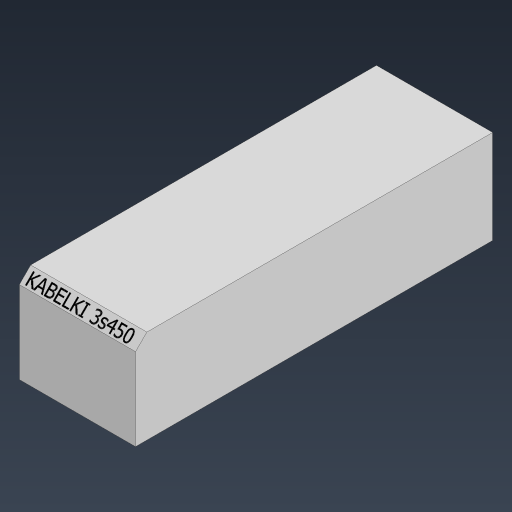
# Autodesk Inventor part: 2s450mah
Saved by Autodesk Inventor 2026.2 (Build 302298010, 298A)
## iProperties
Created: 2026-03-09
Part Number: 2s450mah
Material: Generic
Document SubType Name: Modeling
Designer: szymo
Density: 1 g/cm^3
Appearance: Default
Author: szymo
Autodesk Inventor part; units mm, degrees
ref_plane "YZ Plane" through (0, 0, 0) normal (1, 0, 0) x (0, 1, 0)
ref_plane "XZ Plane" through (0, 0, 0) normal (0, 1, 0) x (-1, 0, 0)
ref_plane "XY Plane" through (0, 0, 0) normal (0, 0, 1) x (1, 0, 0)
sketch "Sketch1" plane through (0, 0, 0) normal (0, 1, 0) x (-1, 0, 0)
  line L0 (0, 0) -> (-20.5, 0)
  line L1 (-20.5, 0) -> (-20.5, -63)
  line L2 (-20.5, -63) -> (0, -63)
  line L3 (0, -63) -> (0, 0)
  dimension "d0" = 20.5
  dimension "d1" = 63
  constraints: 8 end point, 2 parallel, 1 horizontal, 1 perpendicular
  measures "d0" distance of L2.end L1.end
  measures "d1" distance of L0.end L1.end
extrude "Extrusion1" add sketch "Sketch1" along normal blind 16.5
chamfer "Chamfer1" distance 2 angle 45 1 edges at (10.25, 16.5, 0)
sketch "Sketch2" plane through (0, 16.5, -2) normal (0, 0.7071068, 0.7071068) x (1, 0, 0)
  line L0 (0.6017, -0.4664) -> (21.0819, -0.4664) construction
  line L1 (21.0819, -0.4664) -> (21.0819, -2.9145) construction
  line L2 (21.0819, -2.9145) -> (0.6017, -2.9145) construction
  line L3 (0.6017, -2.9145) -> (0.6017, -0.4664) construction
  line L4 (2.263, -2.5085) -> (1.9178, -2.5085)
  line L5 (1.9178, -2.5085) -> (1.1868, -1.5782)
  line L6 (1.1868, -1.5782) -> (1.0701, -1.7095)
  line L7 (1.0701, -1.7095) -> (1.0701, -2.5085)
  line L8 (1.0701, -2.5085) -> (0.8043, -2.5085)
  line L9 (0.8043, -2.5085) -> (0.8043, -0.5085)
  line L10 (0.8043, -0.5085) -> (1.0701, -0.5085)
  line L11 (1.0701, -0.5085) -> (1.0701, -1.4275)
  line L12 (1.0701, -1.4275) -> (1.8902, -0.5085)
  line L13 (1.8902, -0.5085) -> (2.2144, -0.5085)
  line L14 (2.2144, -0.5085) -> (1.3862, -1.4015)
  line L15 (1.3862, -1.4015) -> (2.263, -2.5085)
  line L16 (2.2063, -2.5085) -> (2.8805, -0.5085)
  line L17 (2.8805, -0.5085) -> (3.2079, -0.5085)
  line L18 (3.2079, -0.5085) -> (3.8821, -2.5085)
  line L19 (3.8821, -2.5085) -> (3.6017, -2.5085)
  line L20 (3.6017, -2.5085) -> (3.4202, -1.9493)
  line L21 (3.4202, -1.9493) -> (2.6568, -1.9493)
  line L22 (2.6568, -1.9493) -> (2.4753, -2.5085)
  line L23 (2.4753, -2.5085) -> (2.2063, -2.5085)
  line L24 (3.3473, -1.7224) -> (3.0377, -0.7808)
  line L25 (3.0377, -0.7808) -> (2.7298, -1.7224)
  line L26 (2.7298, -1.7224) -> (3.3473, -1.7224)
  spline S0 degree 2 poles (5.4283, -1.8942) (5.4283, -2.0433) (5.3148, -2.2719) (5.2208, -2.3464) knots 0 0 0 1 2 2 2
  spline S1 degree 2 poles (5.2208, -2.3464) (5.1074, -2.4339) (4.8497, -2.5085) (4.6455, -2.5085) knots 0 0 0 1 2 2 2
  line L27 (4.6455, -2.5085) -> (4.0717, -2.5085)
  line L28 (4.0717, -2.5085) -> (4.0717, -0.5085)
  line L29 (4.0717, -0.5085) -> (4.6017, -0.5085)
  spline S2 degree 2 poles (4.6017, -0.5085) (4.8157, -0.5085) (5.0296, -0.5361) (5.1268, -0.5895) knots 0 0 0 1 2 2 2
  spline S3 degree 2 poles (5.1268, -0.5895) (5.2354, -0.6463) (5.3343, -0.8327) (5.3343, -0.9591) knots 0 0 0 1 2 2 2
  spline S4 degree 2 poles (5.3343, -0.9591) (5.3343, -1.1001) (5.1852, -1.3237) (5.0539, -1.3869) knots 0 0 0 1 2 2 2
  line L30 (5.0539, -1.3869) -> (5.0539, -1.3967)
  spline S5 degree 2 poles (5.0539, -1.3967) (5.2322, -1.4453) (5.4283, -1.703) (5.4283, -1.8942) knots 0 0 0 1 2 2 2
  spline S6 degree 2 poles (5.1512, -1.9056) (5.1512, -1.7921) (5.0863, -1.6463) (4.9891, -1.5944) knots 0 0 0 1 2 2 2
  spline S7 degree 2 poles (4.9891, -1.5944) (4.9259, -1.562) (4.7768, -1.5425) (4.639, -1.5425) knots 0 0 0 1 2 2 2
  line L31 (4.639, -1.5425) -> (4.3375, -1.5425)
  line L32 (4.3375, -1.5425) -> (4.3375, -2.2816)
  line L33 (4.3375, -2.2816) -> (4.5531, -2.2816)
  spline S8 degree 2 poles (4.5531, -2.2816) (4.7281, -2.2816) (4.9291, -2.2492) (5.0069, -2.1973) knots 0 0 0 1 2 2 2
  spline S9 degree 2 poles (5.0069, -2.1973) (5.0815, -2.1438) (5.1512, -2.0109) (5.1512, -1.9056) knots 0 0 0 1 2 2 2
  spline S10 degree 2 poles (5.0571, -0.9963) (5.0571, -0.925) (5.0085, -0.8181) (4.955, -0.7873) knots 0 0 0 1 2 2 2
  spline S11 degree 2 poles (4.955, -0.7873) (4.8902, -0.7516) (4.733, -0.7354) (4.592, -0.7354) knots 0 0 0 1 2 2 2
  line L34 (4.592, -0.7354) -> (4.3375, -0.7354)
  line L35 (4.3375, -0.7354) -> (4.3375, -1.3205)
  line L36 (4.3375, -1.3205) -> (4.639, -1.3205)
  spline S12 degree 2 poles (4.639, -1.3205) (4.7638, -1.3205) (4.8821, -1.2946) (4.9453, -1.254) knots 0 0 0 1 2 2 2
  spline S13 degree 2 poles (4.9453, -1.254) (5.0069, -1.2151) (5.0571, -1.0903) (5.0571, -0.9963) knots 0 0 0 1 2 2 2
  line L37 (5.6925, -2.5085) -> (5.6925, -0.5085)
  line L38 (5.6925, -0.5085) -> (6.9437, -0.5085)
  line L39 (6.9437, -0.5085) -> (6.9437, -0.7451)
  line L40 (6.9437, -0.7451) -> (5.9583, -0.7451)
  line L41 (5.9583, -0.7451) -> (5.9583, -1.2929)
  line L42 (5.9583, -1.2929) -> (6.8772, -1.2929)
  line L43 (6.8772, -1.2929) -> (6.8772, -1.5296)
  line L44 (6.8772, -1.5296) -> (5.9583, -1.5296)
  line L45 (5.9583, -1.5296) -> (5.9583, -2.2719)
  line L46 (5.9583, -2.2719) -> (6.9437, -2.2719)
  line L47 (6.9437, -2.2719) -> (6.9437, -2.5085)
  line L48 (6.9437, -2.5085) -> (5.6925, -2.5085)
  line L49 (8.3943, -2.5085) -> (7.2354, -2.5085)
  line L50 (7.2354, -2.5085) -> (7.2354, -0.5085)
  line L51 (7.2354, -0.5085) -> (7.5012, -0.5085)
  line L52 (7.5012, -0.5085) -> (7.5012, -2.2719)
  line L53 (7.5012, -2.2719) -> (8.3943, -2.2719)
  line L54 (8.3943, -2.2719) -> (8.3943, -2.5085)
  line L55 (10.062, -2.5085) -> (9.7168, -2.5085)
  line L56 (9.7168, -2.5085) -> (8.9858, -1.5782)
  line L57 (8.9858, -1.5782) -> (8.8691, -1.7095)
  line L58 (8.8691, -1.7095) -> (8.8691, -2.5085)
  line L59 (8.8691, -2.5085) -> (8.6033, -2.5085)
  line L60 (8.6033, -2.5085) -> (8.6033, -0.5085)
  line L61 (8.6033, -0.5085) -> (8.8691, -0.5085)
  line L62 (8.8691, -0.5085) -> (8.8691, -1.4275)
  line L63 (8.8691, -1.4275) -> (9.6892, -0.5085)
  line L64 (9.6892, -0.5085) -> (10.0134, -0.5085)
  line L65 (10.0134, -0.5085) -> (9.1852, -1.4015)
  line L66 (9.1852, -1.4015) -> (10.062, -2.5085)
  line L67 (10.9178, -2.5085) -> (10.143, -2.5085)
  line L68 (10.143, -2.5085) -> (10.143, -2.3043)
  line L69 (10.143, -2.3043) -> (10.3975, -2.3043)
  line L70 (10.3975, -2.3043) -> (10.3975, -0.7127)
  line L71 (10.3975, -0.7127) -> (10.143, -0.7127)
  line L72 (10.143, -0.7127) -> (10.143, -0.5085)
  line L73 (10.143, -0.5085) -> (10.9178, -0.5085)
  line L74 (10.9178, -0.5085) -> (10.9178, -0.7127)
  line L75 (10.9178, -0.7127) -> (10.6633, -0.7127)
  line L76 (10.6633, -0.7127) -> (10.6633, -2.3043)
  line L77 (10.6633, -2.3043) -> (10.9178, -2.3043)
  line L78 (10.9178, -2.3043) -> (10.9178, -2.5085)
  spline S14 degree 2 poles (12.5888, -0.6981) (12.5158, -0.6981) (12.3716, -0.7338) (12.3019, -0.7613) knots 0 0 0 1 2 2 2
  spline S15 degree 2 poles (12.3019, -0.7613) (12.2371, -0.7889) (12.1414, -0.8472) (12.1042, -0.8732) knots 0 0 0 1 2 2 2
  line L79 (12.1042, -0.8732) -> (12.0879, -0.8732)
  line L80 (12.0879, -0.8732) -> (12.0879, -0.5895)
  spline S16 degree 2 poles (12.0879, -0.5895) (12.1755, -0.5425) (12.4753, -0.4664) (12.6098, -0.4664) knots 0 0 0 1 2 2 2
  spline S17 degree 2 poles (12.6098, -0.4664) (12.746, -0.4664) (12.9486, -0.5215) (13.0312, -0.5798) knots 0 0 0 1 2 2 2
  spline S18 degree 2 poles (13.0312, -0.5798) (13.1187, -0.643) (13.2095, -0.8262) (13.2095, -0.9493) knots 0 0 0 1 2 2 2
  spline S19 degree 2 poles (13.2095, -0.9493) (13.2095, -1.1147) (12.9923, -1.3643) (12.84, -1.3967) knots 0 0 0 1 2 2 2
  line L81 (12.84, -1.3967) -> (12.84, -1.4161)
  spline S20 degree 2 poles (12.84, -1.4161) (12.9032, -1.4291) (13.0474, -1.4874) (13.109, -1.5458) knots 0 0 0 1 2 2 2
  spline S21 degree 2 poles (13.109, -1.5458) (13.1706, -1.6025) (13.2484, -1.784) (13.2484, -1.9153) knots 0 0 0 1 2 2 2
  spline S22 degree 2 poles (13.2484, -1.9153) (13.2484, -2.0498) (13.156, -2.2784) (13.0717, -2.3659) knots 0 0 0 1 2 2 2
  spline S23 degree 2 poles (13.0717, -2.3659) (12.9842, -2.4566) (12.7362, -2.5506) (12.579, -2.5506) knots 0 0 0 1 2 2 2
  spline S24 degree 2 poles (12.579, -2.5506) (12.4283, -2.5506) (12.1333, -2.4777) (12.0328, -2.4275) knots 0 0 0 1 2 2 2
  line L82 (12.0328, -2.4275) -> (12.0328, -2.1438)
  line L83 (12.0328, -2.1438) -> (12.0523, -2.1438)
  spline S25 degree 2 poles (12.0523, -2.1438) (12.1366, -2.2054) (12.4218, -2.3189) (12.5628, -2.3189) knots 0 0 0 1 2 2 2
  spline S26 degree 2 poles (12.5628, -2.3189) (12.6455, -2.3189) (12.8108, -2.267) (12.8659, -2.207) knots 0 0 0 1 2 2 2
  spline S27 degree 2 poles (12.8659, -2.207) (12.9194, -2.1471) (12.9761, -2.0045) (12.9761, -1.8959) knots 0 0 0 1 2 2 2
  spline S28 degree 2 poles (12.9761, -1.8959) (12.9761, -1.7873) (12.9129, -1.6463) (12.8562, -1.6057) knots 0 0 0 1 2 2 2
  spline S29 degree 2 poles (12.8562, -1.6057) (12.7995, -1.5652) (12.6455, -1.5344) (12.5547, -1.5344) knots 0 0 0 1 2 2 2
  line L84 (12.5547, -1.5344) -> (12.4413, -1.5344)
  line L85 (12.4413, -1.5344) -> (12.4413, -1.3124)
  line L86 (12.4413, -1.3124) -> (12.5304, -1.3124)
  spline S30 degree 2 poles (12.5304, -1.3124) (12.7103, -1.3124) (12.9372, -1.1406) (12.9372, -0.9769) knots 0 0 0 1 2 2 2
  spline S31 degree 2 poles (12.9372, -0.9769) (12.9372, -0.9007) (12.8789, -0.7921) (12.8319, -0.7597) knots 0 0 0 1 2 2 2
  spline S32 degree 2 poles (12.8319, -0.7597) (12.7816, -0.7257) (12.6584, -0.6981) (12.5888, -0.6981) knots 0 0 0 1 2 2 2
  spline S33 degree 2 poles (13.9923, -2.5442) (13.8416, -2.5442) (13.5807, -2.4631) (13.4948, -2.4177) knots 0 0 0 1 2 2 2
  line L87 (13.4948, -2.4177) -> (13.4948, -2.1341)
  line L88 (13.4948, -2.1341) -> (13.5077, -2.1341)
  spline S34 degree 2 poles (13.5077, -2.1341) (13.5401, -2.16) (13.6277, -2.2216) (13.7006, -2.2557) knots 0 0 0 1 2 2 2
  spline S35 degree 2 poles (13.7006, -2.2557) (13.7638, -2.2865) (13.9194, -2.3318) (14.002, -2.3318) knots 0 0 0 1 2 2 2
  spline S36 degree 2 poles (14.002, -2.3318) (14.062, -2.3318) (14.1998, -2.3043) (14.2322, -2.2816) knots 0 0 0 1 2 2 2
  spline S37 degree 2 poles (14.2322, -2.2816) (14.2792, -2.2508) (14.3213, -2.1811) (14.3213, -2.1098) knots 0 0 0 1 2 2 2
  spline S38 degree 2 poles (14.3213, -2.1098) (14.3213, -2.0207) (14.2241, -1.9283) (14.0993, -1.8975) knots 0 0 0 1 2 2 2
  spline S39 degree 2 poles (14.0993, -1.8975) (14.0507, -1.8861) (13.8951, -1.8537) (13.8286, -1.8359) knots 0 0 0 1 2 2 2
  spline S40 degree 2 poles (13.8286, -1.8359) (13.6568, -1.7856) (13.5012, -1.5782) (13.5012, -1.4307) knots 0 0 0 1 2 2 2
  spline S41 degree 2 poles (13.5012, -1.4307) (13.5012, -1.2265) (13.8076, -0.972) (14.0604, -0.972) knots 0 0 0 1 2 2 2
  spline S42 degree 2 poles (14.0604, -0.972) (14.1852, -0.972) (14.438, -1.0336) (14.5239, -1.0806) knots 0 0 0 1 2 2 2
  line L89 (14.5239, -1.0806) -> (14.5239, -1.3513)
  line L90 (14.5239, -1.3513) -> (14.511, -1.3513)
  spline S43 degree 2 poles (14.511, -1.3513) (14.4137, -1.2735) (14.1771, -1.1844) (14.0555, -1.1844) knots 0 0 0 1 2 2 2
  spline S44 degree 2 poles (14.0555, -1.1844) (13.9307, -1.1844) (13.7589, -1.2897) (13.7589, -1.3951) knots 0 0 0 1 2 2 2
  spline S45 degree 2 poles (13.7589, -1.3951) (13.7589, -1.4907) (13.861, -1.5831) (13.9745, -1.6122) knots 0 0 0 1 2 2 2
  spline S46 degree 2 poles (13.9745, -1.6122) (14.0296, -1.6268) (14.169, -1.656) (14.2452, -1.6738) knots 0 0 0 1 2 2 2
  spline S47 degree 2 poles (14.2452, -1.6738) (14.4105, -1.716) (14.579, -1.9088) (14.579, -2.0758) knots 0 0 0 1 2 2 2
  spline S48 degree 2 poles (14.579, -2.0758) (14.579, -2.173) (14.5029, -2.3448) (14.4283, -2.408) knots 0 0 0 1 2 2 2
  spline S49 degree 2 poles (14.4283, -2.408) (14.3489, -2.4745) (14.1463, -2.5442) (13.9923, -2.5442) knots 0 0 0 1 2 2 2
  line L91 (16.0636, -1.8213) -> (15.8254, -1.8213)
  line L92 (15.8254, -1.8213) -> (15.8254, -2.5085)
  line L93 (15.8254, -2.5085) -> (15.5677, -2.5085)
  line L94 (15.5677, -2.5085) -> (15.5677, -1.8213)
  line L95 (15.5677, -1.8213) -> (14.6844, -1.8213)
  line L96 (14.6844, -1.8213) -> (14.6844, -1.5393)
  line L97 (14.6844, -1.5393) -> (15.579, -0.5085)
  line L98 (15.579, -0.5085) -> (15.8254, -0.5085)
  line L99 (15.8254, -0.5085) -> (15.8254, -1.6057)
  line L100 (15.8254, -1.6057) -> (16.0636, -1.6057)
  line L101 (16.0636, -1.6057) -> (16.0636, -1.8213)
  line L102 (15.5677, -1.6057) -> (15.5677, -0.8245)
  line L103 (15.5677, -0.8245) -> (14.8951, -1.6057)
  line L104 (14.8951, -1.6057) -> (15.5677, -1.6057)
  spline S50 degree 2 poles (17.4899, -1.8732) (17.4899, -2.0174) (17.3975, -2.2638) (17.3132, -2.3545) knots 0 0 0 1 2 2 2
  spline S51 degree 2 poles (17.3132, -2.3545) (17.2289, -2.4453) (16.9777, -2.5506) (16.8221, -2.5506) knots 0 0 0 1 2 2 2
  spline S52 degree 2 poles (16.8221, -2.5506) (16.6795, -2.5506) (16.4007, -2.4874) (16.2986, -2.4372) knots 0 0 0 1 2 2 2
  line L105 (16.2986, -2.4372) -> (16.2986, -2.1536)
  line L106 (16.2986, -2.1536) -> (16.3181, -2.1536)
  spline S53 degree 2 poles (16.3181, -2.1536) (16.3489, -2.1762) (16.464, -2.2346) (16.5336, -2.2605) knots 0 0 0 1 2 2 2
  spline S54 degree 2 poles (16.5336, -2.2605) (16.6131, -2.2881) (16.7443, -2.3189) (16.827, -2.3189) knots 0 0 0 1 2 2 2
  spline S55 degree 2 poles (16.827, -2.3189) (16.908, -2.3189) (17.0604, -2.2605) (17.1155, -2.1973) knots 0 0 0 1 2 2 2
  spline S56 degree 2 poles (17.1155, -2.1973) (17.1657, -2.1374) (17.2176, -1.9785) (17.2176, -1.8715) knots 0 0 0 1 2 2 2
  spline S57 degree 2 poles (17.2176, -1.8715) (17.2176, -1.7646) (17.1593, -1.6284) (17.1042, -1.5831) knots 0 0 0 1 2 2 2
  spline S58 degree 2 poles (17.1042, -1.5831) (17.0474, -1.5328) (16.8789, -1.4907) (16.7768, -1.4907) knots 0 0 0 1 2 2 2
  spline S59 degree 2 poles (16.7768, -1.4907) (16.6665, -1.4907) (16.4477, -1.5247) (16.3813, -1.5393) knots 0 0 0 1 2 2 2
  line L107 (16.3813, -1.5393) -> (16.3813, -0.5085)
  line L108 (16.3813, -0.5085) -> (17.4785, -0.5085)
  line L109 (17.4785, -0.5085) -> (17.4785, -0.7435)
  line L110 (17.4785, -0.7435) -> (16.639, -0.7435)
  line L111 (16.639, -0.7435) -> (16.639, -1.2767)
  spline S60 degree 2 poles (16.639, -1.2767) (16.6876, -1.2703) (16.7816, -1.2654) (16.8205, -1.2654) knots 0 0 0 1 2 2 2
  spline S61 degree 2 poles (16.8205, -1.2654) (16.9745, -1.2654) (17.1868, -1.3156) (17.2841, -1.3902) knots 0 0 0 1 2 2 2
  spline S62 degree 2 poles (17.2841, -1.3902) (17.3829, -1.4647) (17.4899, -1.6916) (17.4899, -1.8732) knots 0 0 0 1 2 2 2
  spline S63 degree 2 poles (19.0231, -1.5085) (19.0231, -2.0466) (18.7103, -2.5506) (18.3845, -2.5506) knots 0 0 0 1 2 2 2
  spline S64 degree 2 poles (18.3845, -2.5506) (18.0539, -2.5506) (17.7443, -2.0369) (17.7443, -1.5101) knots 0 0 0 1 2 2 2
  spline S65 degree 2 poles (17.7443, -1.5101) (17.7443, -0.9688) (18.0571, -0.468) (18.3845, -0.468) knots 0 0 0 1 2 2 2
  spline S66 degree 2 poles (18.3845, -0.468) (18.7136, -0.468) (19.0231, -0.9866) (19.0231, -1.5085) knots 0 0 0 1 2 2 2
  spline S67 degree 2 poles (18.6795, -2.1179) (18.7184, -2.019) (18.7508, -1.7143) (18.7508, -1.5085) knots 0 0 0 1 2 2 2
  spline S68 degree 2 poles (18.7508, -1.5085) (18.7508, -1.3027) (18.7184, -0.9996) (18.6779, -0.8975) knots 0 0 0 1 2 2 2
  spline S69 degree 2 poles (18.6779, -0.8975) (18.6374, -0.7954) (18.4964, -0.69) (18.3845, -0.69) knots 0 0 0 1 2 2 2
  spline S70 degree 2 poles (18.3845, -0.69) (18.2727, -0.69) (18.1285, -0.7954) (18.0863, -0.9007) knots 0 0 0 1 2 2 2
  spline S71 degree 2 poles (18.0863, -0.9007) (18.0458, -1.0028) (18.0166, -1.314) (18.0166, -1.5101) knots 0 0 0 1 2 2 2
  spline S72 degree 2 poles (18.0166, -1.5101) (18.0166, -1.7208) (18.0426, -2.0028) (18.0847, -2.113) knots 0 0 0 1 2 2 2
  spline S73 degree 2 poles (18.0847, -2.113) (18.1236, -2.2168) (18.2678, -2.3286) (18.3845, -2.3286) knots 0 0 0 1 2 2 2
  spline S74 degree 2 poles (18.3845, -2.3286) (18.4948, -2.3286) (18.639, -2.2233) (18.6795, -2.1179) knots 0 0 0 1 2 2 2
  point P0 (0, -13.0815)
  constraints: 2 other
extrude "Extrusion2" cut sketch "Sketch2" against normal blind 1
body "Solid1"
